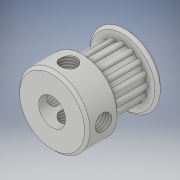
# Autodesk Inventor part: pulley chamfer
Saved by Autodesk Inventor 2019 (Build 230136000, 136)
## iProperties
Created: 2020-02-11
Part Number: pulley chamfer
Material: Generic
Document SubType Name: Modeling
Designer: Vinayak
Density: 1 g/cm^3
Appearance: Default
Author: Vinayak
Autodesk Inventor part; units mm, degrees
ref_plane "YZ Plane" through (0, 0, 0) normal (1, 0, 0) x (0, 1, 0)
ref_plane "XZ Plane" through (0, 0, 0) normal (0, 1, 0) x (-1, 0, 0)
ref_plane "XY Plane" through (0, 0, 0) normal (0, 0, 1) x (1, 0, 0)
sketch "Sketch1" plane through (0, 0, 0) normal (0, 0, 1) x (1, 0, 0)
  circle A0 centre (0, 0) radius 4.3739
  constraints: 1 centre point
extrude "Extrusion1" add sketch "Sketch1" along normal blind 7
sketch "Sketch2" plane through (0, 0, 7) normal (0, 0, 1) x (1, 0, 0)
  circle A0 centre (0, 0) radius 4.3739 projected
  arc A1 (0.4754, 4.348) -> (-0.4754, 4.348) centre (0, 4.3739) ccw
  dimension "d5" = 0.9522
  constraints: 5 point on circle, 1 centre point
  measures "d5" diameter of A1
extrude "Extrusion2" add sketch "Sketch2" against normal blind 7 contours A0 A1
pattern_circular "Circular Pattern1" count 16 over 360 about axis through (0, 0, 0) along (0, 0, 1) of "Extrusion2"
sketch "Sketch3" plane through (0, 0, 7) normal (0, 0, 1) x (1, 0, 0)
  circle A0 centre (0, 0) radius 6.5
  dimension "d11" = 13
  constraints: 1 centre point, 1 coincident
  measures "d11" diameter of A0
extrude "Extrusion3" add sketch "Sketch3" along normal blind 6
sketch "Sketch4" plane through (0, 0, 0) normal (0, 0, -1) x (-1, 0, 0)
  circle A0 centre (0, 0) radius 6.5
  dimension "d14" = 13
  constraints: 1 centre point, 1 coincident
  measures "d14" diameter of A0
extrude "Extrusion4" add sketch "Sketch4" along normal blind 1
sketch "Sketch5" plane through (0, 0, 0) normal (0, 1, 0) x (-1, 0, 0)
  line L0 (0, 0) -> (6, 0)
  dimension "d17" = 6
  constraints: 2 end point, 1 horizontal
  measures "d17" distance of L0.start L0.end
sketch "Sketch6" plane through (0, 0, 0) normal (0, 1, 0) x (-1, 0, 0)
  line L0 (6.5, 13) -> (-6.5, 13) projected
  line L1 (0, 13) -> (0, 7)
  circle A0 centre (0, 10) radius 1.5
  point P0 (0, 0)
  dimension "d18" = 6
  dimension "d19" = 3
  constraints: 2 end point, 2 midpoint, 1 centre point, 1 vertical
  measures "d18" distance of L1.start L1.end
  measures "d19" diameter of A0
extrude "Extrusion5" cut sketch "Sketch6" along normal mid plane 13
pattern_circular "Circular Pattern2" count 4 over 360 about axis through (0, 0, 7) along (0, 0, 1) of "Extrusion5"
thread "Thread1" size "M3x0.5" class "6H" standard "ANSI Metric M Profile" full length
thread "Thread2" size "M3x0.5" class "6H" standard "ANSI Metric M Profile" full length
thread "Thread3" size "M3x0.5" class "6H" standard "ANSI Metric M Profile" full length
thread "Thread4" size "M3x0.5" class "6H" standard "ANSI Metric M Profile" full length
sketch "Sketch7" plane through (0, 0, 13) normal (0, 0, 1) x (1, 0, 0)
  line L0 (0, 0) -> (0, 0) projected
  circle A0 centre (0, 0) radius 2.5
  dimension "d33" = 5
  constraints: 1 centre point, 1 coincident
  measures "d33" diameter of A0
extrude "Extrusion6" cut sketch "Sketch7" against normal blind 14
chamfer "Chamfer1" distance 0.5 angle 45 5 edges at (-6.5, 0, 13) (-6.5, 0, 7) (6.5, 0, 0) (6.5, 0, -1) (-2.5, 0, -1)
body "Solid1"
